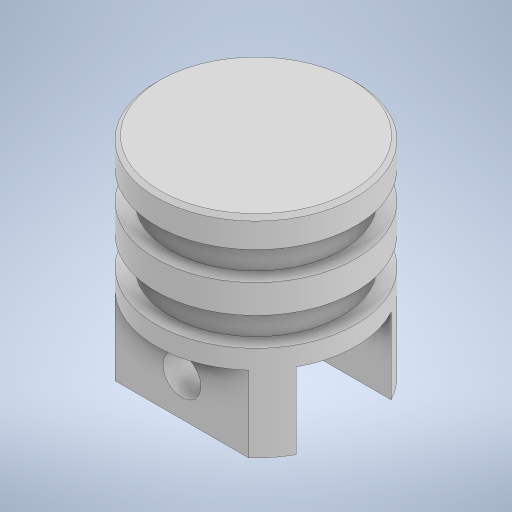
# Autodesk Inventor part: Piston
Saved by Autodesk Inventor 2023 (Build 270158000, 158)
## iProperties
Created: 2022-10-26
Part Number: Piston
Material: Generic
Document SubType Name: Modeling
Designer: tommy
Density: 1 g/cm^3
Appearance: Default
Author: tommy
Autodesk Inventor part; units mm, degrees
ref_plane "YZ Plane" through (0, 0, 0) normal (1, 0, 0) x (0, 1, 0)
ref_plane "XZ Plane" through (0, 0, 0) normal (0, 1, 0) x (-1, 0, 0)
ref_plane "XY Plane" through (0, 0, 0) normal (0, 0, 1) x (1, 0, 0)
sketch "Sketch5" plane through (0, 0, 0) normal (1, 0, 0) x (0, 1, 0)
  line L0 (0, 0) -> (0, -19.05)
  line L1 (0, -19.05) -> (15.875, -19.05)
  line L2 (0, 0) -> (0, -16.6688)
  line L3 (0, -16.6688) -> (15.875, -16.6688)
  line L4 (15.875, -16.6688) -> (15.875, -14.2875)
  line L5 (15.875, -14.2875) -> (20.6375, -14.2875)
  line L6 (20.6375, -14.2875) -> (20.6375, -16.6688)
  line L7 (20.6375, -16.6688) -> (25.4, -16.6688)
  line L8 (25.4, -16.6688) -> (25.4, -14.2875)
  line L9 (25.4, -14.2875) -> (30.1625, -14.2875)
  line L10 (30.1625, -14.2875) -> (30.1625, -16.6688)
  line L11 (30.1625, -16.6688) -> (34.925, -16.6688)
  line L12 (34.925, -16.6688) -> (34.925, 0)
  line L13 (34.925, 0) -> (0, 0)
  dimension "d11" = 19.05
  dimension "d12" = 15.875
  dimension "d14" = 16.6687
  dimension "d15" = 2.3813
  dimension "d16" = 4.7625
  dimension "d17" = 4.7625
  dimension "d18" = 4.7625
  dimension "d19" = 4.7625
  constraints: 28 end point, 7 point on line, 5 perpendicular, 2 parallel, 2 vertical, 1 horizontal
  measures "d11" distance of L0.start L0.end
  measures "d12" distance of L0.end L1.end
  measures "d14" distance of L0.start L2.end
  measures "d15" distance of L3.end L4.end
  measures "d16" distance of L4.end L5.end
  measures "d17" distance of L6.end L7.end
  measures "d18" distance of L8.end L9.end
  measures "d19" distance of L10.end L11.end
revolve "Revolution1" add sketch "Sketch5" angle 360 about axis through (0, 34.925, 0) along (0, -1, 0)
sketch "Sketch6" plane through (0, 0, 0) normal (0, -1, 0) x (1, 0, 0)
  circle A0 centre (0, 0) radius 16.6687 projected
  line L0 (22.672, -7.9375) -> (-28.1087, -7.9375)
  line L1 (22.672, 7.9375) -> (-28.1087, 7.9375)
  line L2 (22.672, -7.9375) -> (-28.1087, -7.9375)
  line L3 (-28.1087, -7.9375) -> (22.672, -7.9375)
  line L4 (22.672, -7.9375) -> (22.672, 7.9375)
  line L5 (22.672, 7.9375) -> (-28.1087, 7.9375)
  line L6 (-28.1087, 7.9375) -> (-28.1087, -7.9375)
  line L7 (0, -12.3825) -> (22.672, -12.3825)
  line L8 (22.672, -12.3825) -> (-30.0751, -12.3825)
  line L9 (-30.0751, -12.3825) -> (-30.0751, -34.2972)
  line L10 (-30.0751, -34.2972) -> (22.672, -34.2972)
  line L11 (22.672, -34.2972) -> (22.672, -12.3825)
  line L12 (0, 12.3825) -> (22.672, 12.3825)
  line L13 (22.672, 12.3825) -> (-30.0751, 12.3825)
  line L14 (-30.0751, 12.3825) -> (-30.0751, 34.2972)
  line L15 (-30.0751, 34.2972) -> (22.672, 34.2972)
  line L16 (22.672, 34.2972) -> (22.672, 12.3825)
  point P0 (-11.1589, 12.3825)
  point P1 (11.1589, 12.3825)
  point P2 (14.6575, 7.9375)
  point P3 (-14.6575, 7.9375)
  point P4 (-14.6575, -7.9375)
  point P5 (14.6575, -7.9375)
  point P6 (11.1589, -12.3825)
  point P7 (-11.1589, -12.3825)
  constraints: 34 end point, 4 horizontal, 4 parallel, 2 perpendicular
chamfer "Chamfer1" distance 0.635 angle 45 1 edges at (0, 34.925, 16.6688)
extrude "Extrusion1" cut sketch "Sketch6" along normal blind 12.7 and the other way blind 12.7 contours A0 L0 L1 | L12 L13 A0 | A0 L13 L14 L15 L16 L12 | L7 L11 L10 L9 L8 A0 | A0 L8 L7
sketch "Sketch7" plane through (11.1589, 0, -12.3825) normal (0, 0, -1) x (-1, 0, 0)
  line L0 (11.1589, 0) -> (11.1589, 12.7)
  line L1 (25.8164, 12.7) -> (-3.4986, 12.7) projected
  circle A0 centre (11.1589, 6.35) radius 3.175
  dimension "d33" = 6.35
  constraints: 2 end point, 2 midpoint, 1 centre point
  measures "d33" diameter of A0
extrude "Extrusion2" cut sketch "Sketch7" against normal blind 31.75
body "Solid3"
